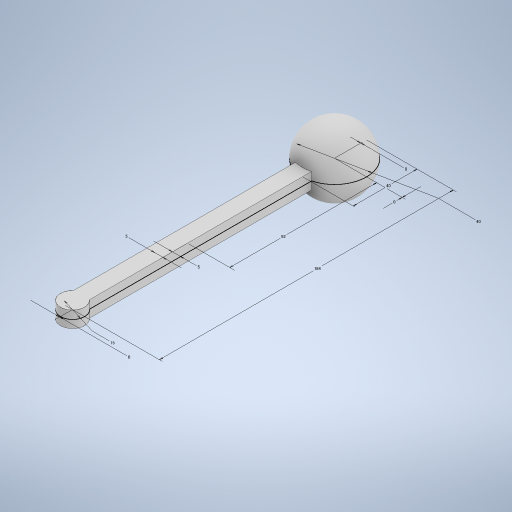
# Autodesk Inventor part: link_kp2heel
Saved by Autodesk Inventor 2024.3 (Build 283343000, 343)
## iProperties
Created: 2025-01-18
Part Number: link_kp2heel
Material: 一般
Document SubType Name: Modeling
Designer: yuu53
Density: 1 g/cm^3
Appearance: 既定
Author: yuu53
Autodesk Inventor part; units mm, degrees
ref_plane "YZ Plane" through (0, 0, 0) normal (1, 0, 0) x (0, 1, 0)
ref_plane "XZ Plane" through (0, 0, 0) normal (0, 1, 0) x (-1, 0, 0)
ref_plane "XY Plane" through (0, 0, 0) normal (0, 0, 1) x (1, 0, 0)
sketch "スケッチ1" plane through (0, 0, 0) normal (0, 1, 0) x (-1, 0, 0)
  line L0 (5, 72) -> (-5, 72)
  line L1 (-5, 72) -> (-5, -92)
  line L2 (-5, -92) -> (5, -92)
  line L3 (5, -92) -> (5, 72)
  circle A0 centre (0, -92) radius 20
  circle A1 centre (0, 72) radius 7.5
  line L4 (0, -112) -> (0, -72)
  point P0 (0, 0)
  point P1 (-5, 66.4098)
  point P2 (-5, -72.6351)
  point P3 (5, -72.6351)
  point P4 (5, 66.4098)
  point P5 (0, -92)
  dimension "d0" = 15
  dimension "d3" = 5
  dimension "d4" = 5
  dimension "d5" = 40
  dimension "d6" = 0
  dimension "d7" = 184
  dimension "d8" = 0
  dimension "d9" = 92
  dimension "d14" = 0
  dimension "d15" = 40
  constraints: 10 end point, 2 centre point, 2 midpoint, 2 parallel, 2 point on circle, 1 horizontal, 1 perpendicular, 1 vertical
  measures "d0" diameter of A1
  measures "d3" distance from line of L1 point (0, 0)
  measures "d4" distance from line of L3 point (0, 0)
  measures "d5" diameter of A0
  measures "d6" distance from line of L2 A0.centre
  measures "d8" distance of point (0, 72) A1.centre
  measures "d9" distance from line of point (0, 0) L2
  measures "d14" distance of point (0, -92) A0.centre
  measures "d15" distance of L4.start L4.end
extrude "押し出し1" add sketch "スケッチ1" along normal blind 5 and the other way blind 5 contours L3 A1 L1 L0 | L0 L1 A1 L3 | L3 A0 L1 A1
revolve "回転1" add sketch "スケッチ1" angle 360 about axis through (0, 0, -112) along (0, 0, 1) contours A0 L4 L2 L3 | L3 L2 L4 A0
